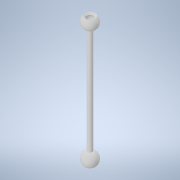
# Autodesk Inventor part: SS_Dyad-01
Saved by Autodesk Inventor 2020.1 (Build 241239000, 239)
## iProperties
Created: 2019-10-24
Part Number: SS_Dyad-01
Material: Generic
Document SubType Name: Modeling
Designer: sshel
Density: 1 g/cm^3
Appearance: Default
Author: sshel
Autodesk Inventor part; units mm, degrees
ref_plane "YZ Plane" through (0, 0, 0) normal (1, 0, 0) x (0, 1, 0)
ref_plane "XZ Plane" through (0, 0, 0) normal (0, 1, 0) x (-1, 0, 0)
ref_plane "XY Plane" through (0, 0, 0) normal (0, 0, 1) x (1, 0, 0)
sketch "Sketch1" plane through (0, 0, 0) normal (0, 1, 0) x (-1, 0, 0)
  line L0 (0, 0) -> (0, -460)
  line L1 (-20, -443.4315) -> (-20, 0)
  arc A0 (-20, -443.4315) -> (-42.4264, -542.4264) centre (0, -500) ccw
  arc A1 (0, -460) -> (-28.2843, -528.2843) centre (0, -500) ccw
  line L2 (-28.2843, -528.2843) -> (-42.4264, -542.4264)
  line L3 (0, 0) -> (-168.1314, 0)
  line L4 (0, 0) -> (0, 460)
  line L5 (-20, 443.4315) -> (-20, 0)
  arc A2 (-42.4264, 542.4264) -> (-20, 443.4315) centre (0, 500) ccw
  arc A3 (-28.2843, 528.2843) -> (0, 460) centre (0, 500) ccw
  line L6 (-28.2843, 528.2843) -> (-42.4264, 542.4264)
  line L7 (0, -759.397) -> (0, 759.397) projected
  dimension "d0" = 20
  dimension "d1" = 20
  dimension "d2" = 45
  dimension "d3" = 40
  dimension "link_length" = 1000
  constraints: 14 end point, 8 point on circle, 6 symmetric about line, 4 centre point, 2 coincident, 2 vertical, 1 horizontal, 1 point on line, 1 vertical alignment, 2 other
  measures "d0" distance between parallel lines of L0 L1
  measures "d1" radial gap between concentric circles of A0 A1
  measures "d2" angle of L3 L2
  measures "d3" radius of A1
  measures "link_length" distance of A3.centre A0.centre
revolve "Revolution1" add sketch "Sketch1" angle 360 about axis through (0, 0, -10) along (0, 0, 1)
equation "\"d0\" = rod_radius"
equation "\"d1\" = rod_radius"
equation "\"d3\" = S_radius"
equation "\"link_length\" = L1"
equation "\"L1\" = 1000"
equation "\"rod_radius\" = 20"
equation "\"S_radius\" = 2 * rod_radius"
equation "\"dyad1_Fx\" = 0"
equation "\"dyad1_Fy\" = 0"
equation "\"dyad1_Fz\" = 0"
equation "\"dyad2_Fy\" = 0"
equation "\"dyad2_Fz\" = 0"
equation "\"dyad3_Fx\" = 0"
equation "\"dyad3_Fz\" = 0"
equation "\"dyad4_Fz\" = 0"
equation "\"dyad5_Fz\" = 0"
body "Solid1"
